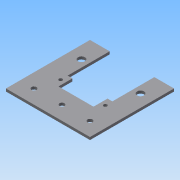
# Autodesk Inventor part: dmc_plate
Saved by Autodesk Inventor 2015 (Build 190159000, 159)
## iProperties
Created: 2014-12-13
Part Number: dmc_plate
Material: Generic
Document SubType Name: Modeling
Designer: Daniel
Density: 1 g/cm^3
Appearance: Default
Author: Daniel
Autodesk Inventor part; units mm, degrees
ref_plane "YZ Plane" through (0, 0, 0) normal (1, 0, 0) x (0, 1, 0)
ref_plane "XZ Plane" through (0, 0, 0) normal (0, 1, 0) x (-1, 0, 0)
ref_plane "XY Plane" through (0, 0, 0) normal (0, 0, 1) x (1, 0, 0)
sketch "Sketch1" plane through (0, 0, 0) normal (0, 1, 0) x (-1, 0, 0)
  line L0 (0, 0) -> (76.2, 0)
  line L1 (76.2, 0) -> (76.2, -76.2)
  line L2 (76.2, -76.2) -> (0, -76.2)
  line L3 (0, -76.2) -> (0, 0)
  dimension "d0" = 76.2
  dimension "d1" = 76.2
  constraints: 8 end point, 2 parallel, 1 horizontal, 1 perpendicular
  measures "d0" distance of L1.end L2.end
  measures "d1" distance of L0.end L1.end
extrude "Extrusion1" add sketch "Sketch1" along normal blind 2.3813
sketch "Sketch2" plane through (0, 2.3813, 0) normal (0, 1, 0) x (1, 0, 0)
  line L0 (-83.8553, 12.7) -> (21.3104, 12.7) construction
  line L1 (-76.2, 0) -> (0, 0) construction
  line L2 (-76.2, 76.2) -> (-76.2, 0) construction
  point P0 (-63.5, 12.7)
  point P1 (-38.1, 12.7)
  point P2 (-12.7, 12.7)
  dimension "d4" = 12.7
  dimension "d5" = 12.7
  dimension "d6" = 25.4
  dimension "d39" = 25.4
  constraints: 3 point on line, 2 end point, 1 horizontal
  measures "d4" distance between parallel lines of L1 L0
  measures "d5" distance from line of point (-63.5, 12.7) L2
  measures "d6" distance of point (-38.1, 12.7) point (-63.5, 12.7)
  measures "d39" distance of point (-12.7, 12.7) point (-38.1, 12.7)
hole "Hole1" at (-63.5, 2.3813, -12.7) at (-38.1, 2.3813, -12.7) at (-12.7, 2.3813, -12.7) direction (0, -1, 0) diameter 4.4958 end through all clearance for "Flat Head Machine Screw (82)" size "#8" standard "Ansi Unified Screw Threads"
sketch "Sketch3" plane through (0, 2.3813, 0) normal (0, 1, 0) x (1, 0, 0)
  line L0 (-85.7811, 31.75) -> (14.4142, 31.75) construction
  line L1 (-76.2, 0) -> (0, 0) construction
  line L2 (-38.1, 80.8292) -> (-38.1, -11.6218) construction
  line L3 (0, 76.2) -> (-76.2, 76.2) construction
  point P0 (-58.3565, 31.75)
  point P1 (-17.8435, 31.75)
  point P2 (-38.1, 76.2)
  dimension "d14" = 31.75
  dimension "d16" = 40.513
  constraints: 4 end point, 3 point on line, 1 horizontal, 1 midpoint, 1 symmetric about line, 1 vertical
  measures "d14" distance between parallel lines of L1 L0
  measures "d16" diameter of point (-58.356, 31.75) L2
hole "Hole2" at (-58.3565, 2.3813, -31.75) at (-17.8435, 2.3813, -31.75) direction (0, -1, 0) diameter 3.175 end through all
sketch "Sketch4" plane through (0, 2.3813, 0) normal (0, 1, 0) x (1, 0, 0)
  line L0 (-58.3565, 76.2) -> (-17.8435, 76.2)
  line L1 (-17.8435, 76.2) -> (-17.8435, 38.1)
  line L2 (-17.8435, 38.1) -> (-58.3565, 38.1)
  line L3 (-58.3565, 38.1) -> (-58.3565, 76.2)
  line L4 (0, 76.2) -> (-76.2, 76.2) projected
  line L5 (-38.1, 81.963) -> (-38.1, -24.4331)
  line L6 (-76.2, 0) -> (0, 0) projected
  line L7 (-53.975, 38.1) -> (-22.225, 38.1)
  line L8 (-22.225, 38.1) -> (-22.225, 25.4)
  line L9 (-22.225, 25.4) -> (-53.975, 25.4)
  line L10 (-53.975, 25.4) -> (-53.975, 38.1)
  point P0 (-38.1, 0)
  dimension "d24" = 38.1
  dimension "d27" = 31.75
  dimension "d28" = 12.7
  dimension "d29" = 40.513
  constraints: 18 end point, 4 parallel, 2 horizontal, 2 perpendicular, 2 point on line, 1 collinear, 1 midpoint, 2 other
  measures "d24" distance between parallel lines of L2 L0
  measures "d27" distance of L8.end L9.end
  measures "d28" distance between parallel lines of L9 L2
  measures "d29" diameter of L3 L5
extrude "Extrusion2" cut sketch "Sketch4" against normal blind 2.3813
sketch "Sketch5" plane through (0, 2.3813, 0) normal (0, 1, 0) x (1, 0, 0)
  line L0 (-81.1122, 57.15) -> (21.0892, 57.15) construction
  line L1 (-58.3565, 76.2) -> (-76.2, 76.2) construction
  line L2 (-38.1, 88.2697) -> (-38.1, -12.0157) construction
  line L3 (-76.2, 0) -> (0, 0) construction
  point P0 (-64.897, 57.15)
  point P1 (-11.303, 57.15)
  point P2 (-38.1, 0)
  dimension "d30" = 19.05
  dimension "d31" = 53.594
  constraints: 4 end point, 3 point on line, 1 horizontal, 1 midpoint, 1 symmetric about line, 1 vertical
  measures "d30" distance between parallel lines of L0 L1
  measures "d31" diameter of point (-64.897, 57.15) L2
hole "Hole3" at (-64.897, 2.3813, -57.15) at (-11.303, 2.3813, -57.15) direction (0, -1, 0) diameter 6.35 end through all
equation "\"d39\" = d6"
body "Solid1"
